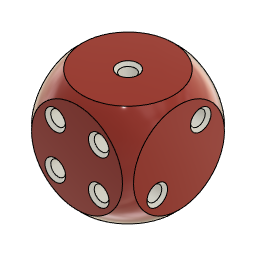
Dice 35 v10 (Autodesk Fusion 360 design; units mm, degrees)
Autodesk Fusion 360 part; units mm, degrees
sketch "Base" plane through (0, 0, 0) normal (0, 0, 1) x (1, 0, 0)
  line L0 (17.5, -17.5) -> (-17.5, -17.5)
  line L1 (-17.5, -17.5) -> (-17.5, 17.5)
  line L2 (-17.5, 17.5) -> (17.5, 17.5)
  line L3 (17.5, 17.5) -> (17.5, -17.5)
  line L4 (17.5, -17.5) -> (-17.5, 17.5) construction
  line L5 (-17.5, -17.5) -> (17.5, 17.5) construction
  dimension "d3" = 35
  dimension "d4" = 35
  constraint horizontal L0
  constraint perpendicular L0 L1
  constraint parallel L0 L2
  constraint parallel L1 L3
  constraint coincident L4 origin
  constraint coincident L5 origin
  measures "d3" distance of L1.end L2.end
  measures "d4" distance of L0.end L1.end
extrude "Extrude1" add sketch "Base" along normal mid plane 35 makes body 1
sphere "SpherePrimitive1" cut diameter 46.9 placed x (0, 1, 0) y (0, 0, 1) z (1, 0, 0) at (0, 0, 0) keep common part bodies 1
sketch "Sketch3" plane through (0, 0, -17.5) normal (0, 0, -1) x (1, 0, 0)
  circle A0 centre (0, 0) radius 15.6094
  circle A1 centre (0, 0) radius 10.5525 construction
  line L0 (-17.5, 17.5) -> (17.5, -17.5) construction
  line L1 (17.5, 17.5) -> (-17.5, -17.5) construction
  point P0 (7.4617, -7.4617)
  point P1 (-7.4617, -7.4617)
  point P2 (-7.4617, 7.4617)
  point P3 (7.4617, 7.4617)
  point P4 (7.4617, 0)
  point P5 (-7.4617, 0)
  dimension "d14" = 21.105
  constraint coincident A0.centre A1.centre
  constraint coincident A1 P0
  constraint coincident L0 P0
  constraint coincident A1 P1
  constraint coincident L1 P1
  constraint coincident A1 P2
  constraint coincident L0 P2
  constraint coincident A1 P3
  constraint coincident L1 P3
  constraint vertical P0 P4
  constraint vertical P1 P5
  constraint horizontal A0.centre P5
  constraint horizontal A0.centre P4
  measures "d14" diameter of A1
sketch "Sketch4" plane through (-17.5, 0, 0) normal (-1, 0, 0) x (0, -1, 0)
  circle A0 centre (0, 0) radius 15.6094
  line L0 (-7.4617, 7.4617) -> (7.4617, 7.4617) construction
  line L1 (7.4617, 7.4617) -> (7.4617, -7.4617) construction
  line L2 (7.4617, -7.4617) -> (-7.4617, -7.4617) construction
  line L3 (-7.4617, -7.4617) -> (-7.4617, 7.4617) construction
  line L4 (-7.4617, 7.4617) -> (7.4617, -7.4617) construction
  line L5 (7.4617, 7.4617) -> (-7.4617, -7.4617) construction
  point P0 (-7.4617, -7.4617)
  point P1 (7.4617, -7.4617)
  point P2 (7.4617, 7.4617)
  point P3 (-7.4617, 7.4617)
  dimension "d15" = 21.105
  constraint horizontal L0
  constraint perpendicular L0 L1
  constraint parallel L0 L2
  constraint parallel L1 L3
  constraint coincident L4 A0.centre
  constraint coincident L5 A0.centre
  constraint coincident A0.centre origin
  constraint equal L2 L3
  constraint coincident P0 L2.end
  constraint coincident P1 L1.end
  constraint coincident P2 L0.end
  constraint coincident P3 L0.start
  measures "d15" distance of P3 P1
sketch "Sketch5" plane through (0, -17.5, 0) normal (0, -1, 0) x (1, 0, 0)
  circle A0 centre (0, 0) radius 15.6094
  line L0 (-7.4617, 7.4617) -> (7.4617, 7.4617) construction
  line L1 (7.4617, 7.4617) -> (7.4617, -7.4617) construction
  line L2 (7.4617, -7.4617) -> (-7.4617, -7.4617) construction
  line L3 (-7.4617, -7.4617) -> (-7.4617, 7.4617) construction
  line L4 (-7.4617, 7.4617) -> (7.4617, -7.4617) construction
  line L5 (7.4617, 7.4617) -> (-7.4617, -7.4617) construction
  point P0 (-7.4617, -7.4617)
  point P1 (7.4617, -7.4617)
  point P2 (7.4617, 7.4617)
  point P3 (-7.4617, 7.4617)
  dimension "d18" = 21.105
  constraint horizontal L0
  constraint perpendicular L0 L1
  constraint parallel L0 L2
  constraint parallel L1 L3
  constraint coincident L4 A0.centre
  constraint coincident L5 A0.centre
  constraint equal L1 L2
  constraint coincident P0 L2.end
  constraint coincident P1 L1.end
  constraint coincident P2 L0.end
  constraint coincident P3 L0.start
  measures "d18" distance of P3 P1
sketch "Sketch6" plane through (0, 17.5, 0) normal (0, 1, 0) x (-1, 0, 0)
  circle A0 centre (0, 0) radius 15.6094
  point P0 (7.4617, 7.4617)
  point P1 (-7.4617, -7.4617)
  point P2 (-7.4617, -7.4617)
  point P3 (7.4617, 7.4617)
  constraint coincident P2 P1
  constraint coincident A0.centre origin
  constraint coincident P3 P0
sketch "Sketch7" plane through (17.5, 0, 0) normal (1, 0, 0) x (0, 1, 0)
  circle A0 centre (0, 0) radius 15.6094
  point P0 (7.4617, 7.4617)
  point P1 (-7.4617, -7.4617)
  point P2 (7.4617, 7.4617)
  point P3 (-7.4617, -7.4617)
  constraint coincident P0 P2
  constraint coincident P1 P3
sketch "Sketch9" plane through (0, 0, 17.5) normal (0, 0, 1) x (-1, 0, 0)
  circle A0 centre (0, 0) radius 15.6094
  constraint coincident A0.centre origin
hole "6 (1)" at (7.4617, 7.4617, -17.5) at (-7.4617, 7.4617, -17.5) at (-7.4617, 0, -17.5) at (-7.4617, -7.4617, -17.5) at (7.4617, -7.4617, -17.5) at (7.4617, 0, -17.5) direction (0, 0, 1) diameter 5.1 depth 6 tip angle 118 countersink diameter 7.1 countersink angle 90 bodies 1
hole "1" at (0, 0, 17.5) direction (0, 0, -1) diameter 5.1 depth 6 tip angle 118 countersink diameter 7.1 countersink angle 90 bodies 1
hole "2 (1)" at (17.5, 7.4617, 7.4617) at (17.5, -7.4617, -7.4617) direction (-1, 0, 0) diameter 5.1 depth 6 tip angle 118 countersink diameter 7.1 countersink angle 90 bodies 1
hole "5 (1)" at (-17.5, -7.4617, -7.4617) at (-17.5, 7.4617, -7.4617) at (-17.5, 0, 0) at (-17.5, 7.4617, 7.4617) at (-17.5, -7.4617, 7.4617) direction (1, 0, 0) diameter 5.1 depth 6 tip angle 118 countersink diameter 7.1 countersink angle 90 bodies 1
hole "3 (1)" at (-7.4617, 17.5, 7.4617) at (7.4617, 17.5, -7.4617) at (0, 17.5, 0) direction (0, -1, 0) diameter 5.1 depth 6 tip angle 118 countersink diameter 7.1 countersink angle 90 bodies 1
hole "4 (1)" at (-7.4617, -17.5, -7.4617) at (-7.4617, -17.5, 7.4617) at (7.4617, -17.5, 7.4617) at (7.4617, -17.5, -7.4617) direction (0, 1, 0) diameter 5.1 depth 6 tip angle 118 countersink diameter 7.1 countersink angle 90 bodies 1
sketch "Pin" plane through (0, 0, 0) normal (0, 0, 1) x (1, 0, 0)
  circle A0 centre (0, 0) radius 2.5
  circle A1 centre (0, 0) radius 3.3
  dimension "d70" = 5
  dimension "d75" = 0.8
  constraint coincident A0.centre A1.centre
  measures "d70" diameter of A0
extrude "Extrude8" add sketch "Pin" along normal blind 5 separate body contours A0 makes body 2
chamfer "Chamfer3" distance 1 angle 45 1 edges at (-2.3308, -0.904, 0) on bodies 2
extrude "Extrude9" add sketch "Pin" along normal blind 0.9 from surface at 5 contours A0 | A1 bodies 2
chamfer "Chamfer4" distance 0.8 angle 45 1 edges at (-3.0767, 1.1933, 5) on bodies 2
equation "w = 35 mm" comment "Strana krychle"
equation "D = w * 1.34" comment "Průměr koule"
equation "d3 = w"
equation "d4 = w"
equation "d5 = w"
equation "d7 = D"
equation "Dh = Dk + 0.1 mm" comment "Průměr otvoru"
equation "k = 0.45" comment "Koeficient rozpěru umístění teček"
equation "d14 = k * D"
equation "d15 = D * k"
equation "d18 = D * k"
equation "h = 6 mm" comment "Hloubka otvoru"
equation "ch = 0.4 mm" comment "Sražení hran otvorů"
equation "Dk = 5 mm" comment "Průměr tečky"
equation "d39 = h"
equation "d40 = Dh"
equation "d42 = Dh + Do"
equation "Do = 2 mm" comment "Osazení otvoru"
equation "d45 = h"
equation "d46 = Dh"
equation "d48 = Dh + Do"
equation "d50 = h"
equation "d51 = Dh"
equation "d53 = Dh + Do"
equation "d55 = h"
equation "d56 = Dh"
equation "d58 = Dh + Do"
equation "d60 = h"
equation "d61 = Dh"
equation "d63 = Dh + Do"
equation "d65 = h"
equation "d66 = Dh"
equation "d68 = Dh + Do"
equation "d70 = Dk"
equation "d71 = h - 0.5 * Do"
equation "d75 = Do / 2.5"
equation "d77 = Do - 1.1 mm"
equation "d79 = Do / 2.5"
named bodies: "D35", "Pin 21x"
